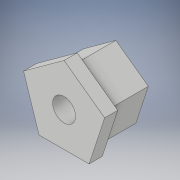
# Autodesk Inventor part: gearNotch
Saved by Autodesk Inventor 2019.1 (Build 231200000, 200)
## iProperties
Created: 2018-12-01
Part Number: gearNotch
Material: Generisch
Document SubType Name: Modeling
Designer: JochenAlt
Density: 1 g/cm^3
Appearance: Vorgabe
Author: JochenAlt
Autodesk Inventor part; units mm, degrees
ref_plane "YZ Plane" through (0, 0, 0) normal (1, 0, 0) x (0, 1, 0)
ref_plane "XZ Plane" through (0, 0, 0) normal (0, 1, 0) x (-1, 0, 0)
ref_plane "XY Plane" through (0, 0, 0) normal (0, 0, 1) x (1, 0, 0)
sketch "Skizze1" plane through (0, 0, 0) normal (0, 0, 1) x (1, 0, 0)
  circle A0 centre (0, 0) radius 3.7 construction
  line L0 (0, 3.7) -> (3.5189, 1.1434)
  line L1 (3.5189, 1.1434) -> (2.1748, -2.9934)
  line L2 (2.1748, -2.9934) -> (-2.1748, -2.9934)
  line L3 (-2.1748, -2.9934) -> (-3.5189, 1.1434)
  line L4 (-3.5189, 1.1434) -> (0, 3.7)
  circle A1 centre (0, 0) radius 5.2 construction
  line L5 (0, 5.2) -> (4.9455, 1.6069)
  line L6 (4.9455, 1.6069) -> (3.0565, -4.2069)
  line L7 (3.0565, -4.2069) -> (-3.0565, -4.2069)
  line L8 (-3.0565, -4.2069) -> (-4.9455, 1.6069)
  line L9 (-4.9455, 1.6069) -> (0, 5.2)
  circle A2 centre (0, 0) radius 1.75
  circle A3 centre (0, 0) radius 6.5 construction
  line L10 (-6.1819, 2.0086) -> (0, 6.5)
  line L11 (0, 6.5) -> (6.1819, 2.0086)
  line L12 (6.1819, 2.0086) -> (3.8206, -5.2586)
  line L13 (3.8206, -5.2586) -> (-3.8206, -5.2586)
  line L14 (-3.8206, -5.2586) -> (-6.1819, 2.0086)
  circle A4 centre (0, 0) radius 4.2 construction
  line L15 (0, 9.1) -> (0, -9.1) construction
  circle A5 centre (0, 0) radius 5.7 construction
  dimension "d9" = 13
  dimension "d8" = 3.5
  dimension "d14" = 8.4
  dimension "d15" = 0.5
  dimension "d16" = 11.4
  dimension "d18" = 0.5
  constraints: 30 end point, 8 coincident, 3 centre point, 2 parallel, 2 vertical alignment, 1 point on line, 40 other
  measures "d8" diameter of A2
  measures "d14" diameter of A4
  measures "d16" diameter of A5
extrude "Extrusion1" add sketch "Skizze1" along normal blind 4.4 contours L5 L6 L7 L8 L9
extrude "Extrusion2" add sketch "Skizze1" along normal blind 1.5 from surface at 4.4 contours L0 L1 L2 L3 L4 | L5 L6 L7 L8 L9
extrude "Extrusion3" add sketch "Skizze1" along normal blind 2 from surface at 5.9 contours L0 L1 L2 L3 L4 | L5 L6 L7 L8 L9 | L10 L11 L12 L13 L14
